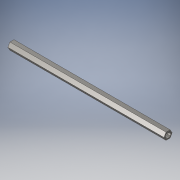
# Autodesk Inventor part: Axle
Saved by Autodesk Inventor 2017 (Build 210142000, 142)
## iProperties
Created: 2017-01-16
Part Number: Axle
Material: Steel, Alloy
Document SubType Name: Modeling
Designer: mmarkle
Density: 7.73 g/cm^3
Appearance: Semi-Polished
Mass: 191.977 g
Surface Area: 81.0151 cm^2
Volume: 24.8353 cm^3
Author: mmarkle
Autodesk Inventor part; units mm, degrees
ref_plane "YZ Plane" through (0, 0, 0) normal (1, 0, 0) x (0, 1, 0)
ref_plane "XZ Plane" through (0, 0, 0) normal (0, 1, 0) x (-1, 0, 0)
ref_plane "XY Plane" through (0, 0, 0) normal (0, 0, 1) x (1, 0, 0)
sketch "Sketch1" plane through (0, 0, 0) normal (1, 0, 0) x (0, 1, 0)
  line L0 (6.35, -3.6662) -> (0, -7.3323)
  line L1 (0, -7.3323) -> (-6.35, -3.6662)
  line L2 (-6.35, -3.6662) -> (-6.35, 3.6662)
  line L3 (-6.35, 3.6662) -> (0, 7.3323)
  line L4 (0, 7.3323) -> (6.35, 3.6662)
  line L5 (6.35, 3.6662) -> (6.35, -3.6662)
  point P0 (0, 0)
  point P1 (0, 0)
  dimension "d3" = 6.35
  constraints: 12 end point, 1 coincident, 13 other
  measures "d3" distance from line of L5 point (0, 0)
extrude "Extrusion1" add sketch "Sketch1" along normal blind 279.4
sketch "Sketch2" plane through (279.4, 0, 0) normal (1, 0, 0) x (0, 0, -1)
  circle A0 centre (0, 0) radius 5.0038
  line L0 (-1.9939, 4.5894) -> (-1.9939, 3.0146)
  line L1 (-1.9939, 3.0146) -> (1.9939, 3.0146)
  line L2 (1.9939, 3.0146) -> (1.9939, 4.5894)
  dimension "d6" = 5.0038
  dimension "d7" = 3.9878
  dimension "d8" = 1.9939
  dimension "d9" = 1.5748
  dimension "d10" = 1.5748
  constraints: 6 end point, 2 point on circle, 1 centre point, 1 coincident, 1 perpendicular, 1 vertical
  measures "d6" radius of A0
  measures "d7" distance of L0.end L1.end
  measures "d8" distance from line of point (0, 0) L0
  measures "d9" distance of L0.start L0.end
  measures "d10" distance of L1.end L2.end
extrude "Extrusion2" cut sketch "Sketch2" against normal through all contours A0 L0 L1 L2 picked at (-0.1705, 0.3505)
body "Solid1"
